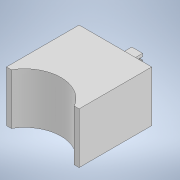
# Autodesk Inventor part: Auswurf_Rampe
Saved by Autodesk Inventor 2020.3 (Build 243373000, 373)
## iProperties
Created: 2021-08-11
Part Number: Auswurf_Rampe
Material: Generisch
Document SubType Name: Modeling
Designer: Preuß P. Ch.
Density: 1 g/cm^3
Appearance: Vorgabe
Author: Preuß P. Ch.
Autodesk Inventor part; units mm, degrees
ref_plane "YZ Plane" through (0, 0, 0) normal (1, 0, 0) x (0, 1, 0)
ref_plane "XZ Plane" through (0, 0, 0) normal (0, 1, 0) x (-1, 0, 0)
ref_plane "XY Plane" through (0, 0, 0) normal (0, 0, 1) x (1, 0, 0)
sketch "Skizze1" plane through (0, 0, 0) normal (0, 0, 1) x (1, 0, 0)
  line L0 (-100, 0) -> (100, 0)
  line L1 (100, 0) -> (100, 140)
  line L2 (100, 140) -> (-100, 140)
  line L3 (-100, 140) -> (-100, 0)
  point P0 (0, 0)
  dimension "d0" = 200
  dimension "d1" = 140
  constraints: 8 end point, 2 parallel, 1 horizontal, 1 perpendicular
  measures "d0" distance of L2.end L1.end
  measures "d1" distance of L1.end L0.end
extrude "Extrusion1" add sketch "Skizze1" along normal blind 200
sketch "Skizze2" plane through (-100, 140, 0) normal (0, 1, 0) x (1, 0, 0)
  circle A0 centre (100, -250) radius 100
  point P0 (100, 0)
  dimension "d4" = 200
  constraints: 1 centre point
  measures "d4" diameter of A0
extrude "Extrusion2" cut sketch "Skizze2" against normal blind 140
sketch "Skizze3" plane through (0, 0, 0) normal (0, 0, -1) x (-1, 0, 0)
  point P0 (0, 0)
sketch "Skizze4" plane through (0, 0, 0) normal (0, 0, -1) x (-1, 0, 0)
  line L0 (15, 68) -> (-15, 68)
  line L1 (-15, 68) -> (-15, 60)
  line L2 (-15, 60) -> (15, 60)
  line L3 (15, 60) -> (15, 68)
  line L4 (-15, 76) -> (15, 76)
  line L5 (15, 76) -> (15, 84)
  line L6 (15, 84) -> (-15, 84)
  line L7 (-15, 84) -> (-15, 76)
  line L8 (-15, 92) -> (15, 92)
  line L9 (15, 92) -> (15, 100)
  line L10 (15, 100) -> (-15, 100)
  line L11 (-15, 100) -> (-15, 92)
  point P0 (0, 0)
  dimension "d7" = 30
  dimension "d8" = 8
  dimension "d9" = 30
  dimension "d10" = 8
  dimension "d11" = 8
  constraints: 24 end point, 6 parallel, 3 horizontal, 3 perpendicular, 1 point on line
  measures "d7" distance of L2.end L1.end
  measures "d8" distance of L1.end L0.end
  measures "d9" distance of L6.end L5.end
  measures "d10" distance of L5.end L4.end
  measures "d11" distance of L9.end L8.end
extrude "Extrusion3" add sketch "Skizze4" along normal blind 60
sketch "Skizze5" plane through (-15, 100, 0) normal (0, 1, 0) x (1, 0, 0)
  circle A0 centre (15, 30) radius 7
  line L0 (0, 60) -> (30, 60) projected
  arc A1 (30, 60) -> (0, 60) centre (15, 60) ccw
  point P0 (15, 0)
  dimension "d14" = 14
  dimension "d15" = 15
  constraints: 2 centre point, 2 point on circle
  measures "d14" diameter of A0
  measures "d15" radius of A1
extrude "Extrusion4" cut sketch "Skizze5" against normal blind 40 contours A0
